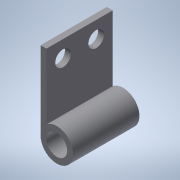
# Autodesk Inventor part: SP29V1 Bisagra P1
Saved by Autodesk Inventor 2021.2 (Build 252289000, 289)
## iProperties
Created: 2026-08-14
Part Number: SP29V1 Bisagra P1
Material: Generic
Document SubType Name: Modeling
Designer: nelso
Density: 1 g/cm^3
Appearance: Default
Author: nelso
Autodesk Inventor part; units mm, degrees
ref_plane "YZ Plane" through (0, 0, 0) normal (1, 0, 0) x (0, 1, 0)
ref_plane "XZ Plane" through (0, 0, 0) normal (0, 1, 0) x (-1, 0, 0)
ref_plane "XY Plane" through (0, 0, 0) normal (0, 0, 1) x (1, 0, 0)
sketch "Sketch1" plane through (0, 0, 0) normal (0, 1, 0) x (-1, 0, 0)
  circle A0 centre (0, 0) radius 3.875
  circle A1 centre (0, 0) radius 4.375
  circle A2 centre (0, 0) radius 6.875
  line L0 (6.875, 0) -> (6.875, 33)
  line L1 (6.875, 33) -> (4.375, 33)
  line L2 (4.375, 33) -> (4.375, 5.3033)
  dimension "d0" = 7.75
  dimension "d1" = 8.75
  dimension "d2" = 13.75
  dimension "d3" = 33
  dimension "d4" = 2.5
  constraints: 6 end point, 3 centre point, 3 coincident, 2 point on circle, 2 vertical, 1 horizontal, 1 tangent
  measures "d0" diameter of A0
  measures "d1" diameter of A1
  measures "d2" diameter of A2
  measures "d3" distance of L0.start L0.end
  measures "d4" distance of L0.end L1.end
extrude "Extrusion1" add sketch "Sketch1" along normal blind 28 contours A2 | A2 L2 L1 L0
sketch "Sketch4" plane through (-4.375, 0, 33) normal (1, 0, 0) x (0, 0, -1)
  line L0 (0, 28) -> (27.6967, 28) projected
  line L1 (0, 0) -> (0, 28) projected
  line L2 (0, 14) -> (27.6967, 14)
  line L3 (0, 14) -> (7, 14)
  line L4 (7, 14) -> (7, 7)
  line L5 (7, 14) -> (7, 21)
  point P0 (33, 0)
  dimension "d7" = 14
  dimension "d17" = 7
  dimension "d18" = 7
  dimension "d19" = 7
  constraints: 8 end point, 1 horizontal, 1 midpoint, 1 perpendicular, 1 point on line, 1 vertical
  measures "d7" distance of L0.start L2.start
  measures "d17" distance of L2.start L3.end
  measures "d18" distance of L3.end L4.end
  measures "d19" distance of L3.end L5.end
hole "Hole1" at (-4.375, 7, 26) at (-4.375, 21, 26) direction (-1, 0, 0) diameter 6.6 end up to face face through (-6.875, 9.3333, 22) facing (-1, 0, 0) clearance for "Countersunk Flat Head Screw ISO 2009/7046" size "M6" standard "ISO"
body "Solid1"
